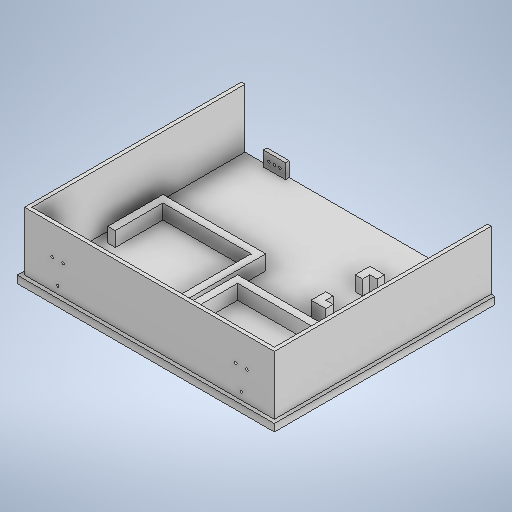
# Autodesk Inventor part: Venstre_bottom
Saved by Autodesk Inventor 2025.2 (Build 292293000, 293)
## iProperties
Created: 2025-05-13
Part Number: Venstre_bottom
Material: Generic
Document SubType Name: Modeling
Designer: lauri
Density: 1 g/cm^3
Appearance: Default
Author: lauri
Autodesk Inventor part; units mm, degrees
ref_plane "YZ Plane" through (0, 0, 0) normal (1, 0, 0) x (0, 1, 0)
ref_plane "XZ Plane" through (0, 0, 0) normal (0, 1, 0) x (-1, 0, 0)
ref_plane "XY Plane" through (0, 0, 0) normal (0, 0, 1) x (1, 0, 0)
sketch "Sketch1" plane through (0, 0, 0) normal (0, 1, 0) x (-1, 0, 0)
  line L0 (-175, 150) -> (175, 150)
  line L1 (175, 150) -> (175, -150)
  line L2 (175, -150) -> (-175, -150)
  line L3 (-175, -150) -> (-175, 150)
  line L4 (-175, 150) -> (175, -150) construction
  line L5 (175, 150) -> (-175, -150) construction
  point P0 (0, 0)
  dimension "d0" = 350
  dimension "d1" = 300
  constraints: 12 end point, 2 midpoint, 2 parallel, 1 horizontal, 1 perpendicular
  measures "d0" distance of L1.end L2.end
  measures "d1" distance of L0.end L1.end
extrude "Extrusion1" add sketch "Sketch1" along normal blind 10
sketch "Sketch2" plane through (0, 10, 0) normal (0, 1, 0) x (1, 0, 0)
  line L0 (175, 150) -> (-175, 150) projected
  line L1 (-175, 150) -> (-170, 150)
  line L2 (-170, 150) -> (-165, 150)
  line L3 (-165, 150) -> (-165, -145)
  line L4 (-165, -145) -> (-170, -145)
  line L5 (-170, -145) -> (-170, 150)
  line L6 (-170, -145) -> (170, -145)
  line L7 (170, -145) -> (170, -140)
  line L8 (170, -140) -> (-170, -140)
  line L9 (-170, -140) -> (-170, -145)
  line L10 (170, -140) -> (165, -140)
  line L11 (165, -140) -> (165, 150)
  line L12 (165, 150) -> (170, 150)
  line L13 (170, 150) -> (170, -140)
  point P0 (0, 0)
  point P1 (-170, 145)
  point P2 (170, 145)
  point P3 (-165, -140)
  point P4 (-165, -145)
  dimension "d5" = 5
  dimension "d6" = 5
  dimension "d7" = 5
  constraints: 26 end point, 6 parallel, 3 horizontal, 3 perpendicular, 2 point on line
  measures "d5" distance of L3.end L4.end
  measures "d6" distance of L7.end L6.end
  measures "d7" distance of L11.end L12.end
extrude "Extrusion2" add sketch "Sketch2" along normal blind 80 contours L13 L8 L11 L0 | L7 L6 L3 L8 | L3 L8 L5 L0 | L3 L4 L5 L8
sketch "Sketch3" plane through (-175, 0, 150) normal (0, 0, 1) x (1, 0, 0)
  line L0 (5, 10) -> (5, 90) projected
  line L1 (5, 90) -> (50, 90)
  line L2 (340, 90) -> (10, 90) projected
  line L3 (50, 90) -> (50, 20)
  line L4 (345, 10) -> (345, 90) projected
  line L5 (345, 90) -> (300, 90)
  line L6 (300, 90) -> (300, 20)
  line L7 (350, 10) -> (345, 10) projected
  line L8 (350, 10) -> (350, 90)
  point P0 (175, 0)
  point P1 (307.5, 50)
  point P2 (292.5, 50)
  point P3 (42.5, 50)
  point P4 (57.5, 50)
  dimension "d10" = 45
  dimension "d11" = 70
  dimension "d12" = 45
  dimension "d13" = 70
  constraints: 10 end point, 2 coincident, 2 point on line, 2 vertical, 1 perpendicular
  measures "d10" distance of L0.end L1.end
  measures "d11" distance of L1.end L3.end
  measures "d12" distance of L4.end L5.end
  measures "d13" distance of L5.end L6.end
sketch "Sketch4" plane through (0, 10, 0) normal (0, 1, 0) x (1, 0, 0)
  line L0 (165, 150) -> (-165, 150) projected
  line L1 (-165, 150) -> (-135, 150)
  line L2 (-135, 150) -> (-105, 150)
  line L3 (-105, 150) -> (-105, 145)
  line L4 (-105, 145) -> (-135, 145)
  line L5 (-135, 145) -> (-135, 150)
  line L6 (165, 150) -> (135, 150)
  line L7 (135, 150) -> (105, 150)
  line L8 (105, 150) -> (105, 145)
  line L9 (105, 145) -> (135, 145)
  line L10 (135, 145) -> (135, 150)
  point P0 (0, 0)
  dimension "d21" = 30
  dimension "d22" = 30
  dimension "d23" = 5
  dimension "d24" = 30
  dimension "d25" = 30
  dimension "d26" = 5
  constraints: 20 end point, 4 parallel, 2 horizontal, 2 perpendicular, 2 point on line
  measures "d21" distance of L0.end L1.end
  measures "d22" distance of L3.end L4.end
  measures "d23" distance of L2.end L3.end
  measures "d24" distance of L0.start L6.end
  measures "d25" distance of L9.end L8.end
  measures "d26" distance of L8.end L7.end
extrude "Extrusion3" add sketch "Sketch4" along normal blind 20
sketch "Sketch5" plane through (175, 0, -150) normal (0, 0, -1) x (-1, 0, 0)
  circle A0 centre (295, 20) radius 1.75 projected
  line L0 (287.5, 20) -> (295, 20)
  point P0 (175, 0)
  point P1 (302.5, 20)
  point P2 (55, 20)
  point P3 (62.5, 20)
  point P4 (47.5, 20)
  dimension "d45" = 7.5
  constraints: 2 coincident, 2 end point, 1 horizontal
  measures "d45" distance of L0.start L0.end
hole "Hole2" at (-120, 20, -150) at (-127.5, 20, -150) at (-112.5, 20, -150) at (120, 20, -150) at (112.5, 20, -150) at (127.5, 20, -150) direction (0, 0, 1) diameter 3.5 depth 10
hole "Hole3" at (-125, 20, 150) at (125, 20, 150) at (132.5, 50, 150) at (117.5, 50, 150) at (-132.5, 50, 150) at (-117.5, 50, 150) direction (0, 0, -1) diameter 3.5 depth 10
sketch "Sketch6" plane through (0, 10, 0) normal (0, 1, 0) x (1, 0, 0)
  line L0 (-165, -140) -> (165, -140) projected
  line L1 (165, -140) -> (215, -140) construction
  line L2 (-5.3553, -129.6447) -> (154.6447, -129.6447)
  line L3 (154.6447, -129.6447) -> (154.6447, -19.6447)
  line L4 (154.6447, -19.6447) -> (-5.3553, -19.6447)
  line L5 (-5.3553, -19.6447) -> (-5.3553, -129.6447)
  line L6 (-5.3553, -129.6447) -> (154.6447, -19.6447) construction
  line L7 (154.6447, -129.6447) -> (-5.3553, -19.6447) construction
  line L8 (4.6447, -119.6447) -> (144.6447, -119.6447)
  line L9 (144.6447, -119.6447) -> (144.6447, -29.6447)
  line L10 (144.6447, -29.6447) -> (4.6447, -29.6447)
  line L11 (4.6447, -29.6447) -> (4.6447, -119.6447)
  line L12 (4.6447, -119.6447) -> (144.6447, -29.6447) construction
  line L13 (144.6447, -119.6447) -> (4.6447, -29.6447) construction
  point P0 (0, 0)
  point P1 (74.6447, -74.6447)
  dimension "d51" = 160
  dimension "d52" = 110
  dimension "d70" = 140
  dimension "d71" = 90
  constraints: 26 end point, 4 parallel, 3 horizontal, 3 midpoint, 2 perpendicular
  measures "d51" distance of L4.end L3.end
  measures "d52" distance of L3.end L2.end
  measures "d70" distance of L10.end L9.end
  measures "d71" distance of L9.end L8.end
sketch "Sketch7" plane through (0, 10, 0) normal (0, 1, 0) x (1, 0, 0)
  line L0 (-165, -140) -> (165, -140) projected
  line L1 (-165, -140) -> (-150.8579, -125.8579)
  line L2 (-165, -140) -> (-145, -140) construction
  line L3 (-150.8579, -125.8579) -> (-10.8579, -125.8579)
  line L4 (-10.8579, -125.8579) -> (-10.8579, 24.1421)
  line L5 (-10.8579, 24.1421) -> (-150.8579, 24.1421)
  line L6 (-150.8579, 24.1421) -> (-150.8579, -125.8579)
  line L7 (-150.8579, -50.8579) -> (-80.8579, -50.8579)
  line L8 (-140.8579, -115.8579) -> (-20.8579, -115.8579)
  line L9 (-20.8579, -115.8579) -> (-20.8579, 14.1421)
  line L10 (-20.8579, 14.1421) -> (-140.8579, 14.1421)
  line L11 (-140.8579, 14.1421) -> (-140.8579, -115.8579)
  line L12 (-140.8579, -115.8579) -> (-20.8579, 14.1421) construction
  line L13 (-20.8579, -115.8579) -> (-140.8579, 14.1421) construction
  line L14 (-140.8579, -115.8579) -> (-150.8579, -115.8579)
  line L15 (-5.3553, -19.6447) -> (154.6447, -19.6447) projected
  line L16 (154.6447, -19.6447) -> (154.6447, 0.3553)
  line L17 (154.6447, 0.3553) -> (74.6447, 0.3553)
  line L18 (74.6447, 0.3553) -> (74.6447, 80.3553)
  line L19 (74.6447, 80.3553) -> (154.6447, 80.3553)
  line L20 (154.6447, 80.3553) -> (154.6447, 0.3553)
  line L21 (84.6447, 70.3553) -> (144.6447, 70.3553)
  line L22 (144.6447, 70.3553) -> (144.6447, 10.3553)
  line L23 (144.6447, 10.3553) -> (84.6447, 10.3553)
  line L24 (84.6447, 10.3553) -> (84.6447, 70.3553)
  line L25 (84.6447, 70.3553) -> (144.6447, 10.3553) construction
  line L26 (144.6447, 70.3553) -> (84.6447, 10.3553) construction
  line L27 (94.645, 70.3553) -> (134.645, 70.3553)
  line L28 (134.645, 70.3553) -> (134.645, 80.3553)
  line L29 (94.645, 80.3553) -> (94.645, 70.3553)
  line L30 (94.645, 10.3553) -> (134.645, 10.3553)
  line L31 (134.645, 0.3553) -> (94.645, 0.3553)
  line L32 (94.645, 80.3553) -> (134.645, 80.3553)
  line L33 (94.645, 10.3553) -> (94.645, 0.3553)
  line L34 (134.645, 10.3553) -> (94.645, 10.3553)
  line L35 (134.645, 10.3553) -> (134.645, 0.3553)
  line L36 (94.645, 0.3553) -> (134.645, 0.3553)
  line L37 (84.6447, 60.355) -> (84.6447, 20.355)
  line L38 (84.6447, 20.355) -> (74.6447, 20.355)
  line L39 (74.6447, 60.355) -> (84.6447, 60.355)
  point P0 (0, 0)
  point P1 (-140.8579, -50.8579)
  point P2 (114.6447, 40.3553)
  dimension "d55" = 20
  dimension "d56" = 45
  dimension "d57" = 140
  dimension "d58" = 150
  dimension "d59" = 120
  dimension "d60" = 130
  dimension "d61" = 20
  dimension "d62" = 80
  dimension "d63" = 80
  dimension "d75" = 60
  dimension "d76" = 60
  dimension "d77" = 40
  dimension "d78" = 40
  constraints: 76 end point, 13 point on line, 10 parallel, 10 perpendicular, 7 horizontal, 5 midpoint, 2 vertical, 1 equal length
  measures "d55" distance of L0.start L1.end
  measures "d56" angle of L2 L1
  measures "d57" distance of L5.end L4.end
  measures "d58" distance of L4.end L3.end
  measures "d59" distance of L10.end L9.end
  measures "d60" distance of L9.end L8.end
  measures "d61" distance of L15.end L16.end
  measures "d62" distance of L18.end L19.end
  measures "d63" distance of L17.end L18.end
  measures "d75" distance of L22.end L23.end
  measures "d76" distance of L21.end L22.end
  measures "d77" distance of L27.start L27.end
  measures "d78" distance of L37.start L37.end
extrude "Extrusion6" add sketch "Sketch6" along normal blind 20
extrude "Extrusion7" add sketch "Sketch7" along normal blind 20 contours L6 L14 L8 L9 L10 L11 L7 L5 L4 L3 | L17 L35 L23 L22 L21 L28 L19 L20 | L17 L18 L38 L24 L23 L33 | L29 L21 L24 L39 L18 L19
body "Solid1"
